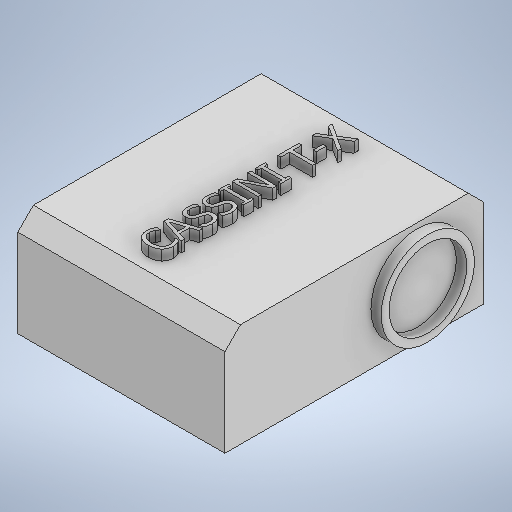
# Autodesk Inventor part: Caméra
Saved by Autodesk Inventor 2026.2 (Build 302298010, 298A)
## iProperties
Created: 2026-04-02
Part Number: Caméra
Material: Générique
Document SubType Name: Modeling
Designer: Genon
Density: 1 g/cm^3
Appearance: Par défaut
Author: Genon
Autodesk Inventor part; units mm, degrees
ref_plane "YZ Plane" through (0, 0, 0) normal (1, 0, 0) x (0, 1, 0)
ref_plane "XZ Plane" through (0, 0, 0) normal (0, 1, 0) x (-1, 0, 0)
ref_plane "XY Plane" through (0, 0, 0) normal (0, 0, 1) x (1, 0, 0)
sketch "Esquisse1" plane through (0, 0, 0) normal (0, 1, 0) x (-1, 0, 0)
  line L0 (0, 0) -> (40, 0)
  line L1 (40, 0) -> (40, -50)
  line L2 (40, -50) -> (0, -50)
  line L3 (0, -50) -> (0, 0)
  dimension "d0" = 40
  dimension "d1" = 50
  constraints: 8 end point, 2 parallel, 1 horizontal, 1 perpendicular
  measures "d0" distance of L1.end L2.end
  measures "d1" distance of L0.end L1.end
extrude "Extrusion1" add sketch "Esquisse1" along normal blind 20
chamfer "Chanfrein1" distance 3 angle 45 2 edges at (-20, 20, 0) (-20, 20, -50)
sketch "Esquisse2" plane through (0, 0, 0) normal (1, 0, 0) x (0, 0, -1)
  circle A0 centre (37.194, 10) radius 7.5
  circle A1 centre (37.194, 10) radius 9
  line L0 (47, 20) -> (3, 20) projected
  line L1 (37.194, 20) -> (37.194, 10)
  line L2 (37.194, 20) -> (47.194, 20) construction
  point P0 (0, 0)
  dimension "d7" = 15
  dimension "d8" = 18
  dimension "d9" = 10
  dimension "d10" = 90
  constraints: 4 end point, 2 centre point, 2 coincident, 2 perpendicular, 1 horizontal, 1 point on line
  measures "d7" diameter of A0
  measures "d8" diameter of A1
  measures "d9" distance of L1.start L1.end
  measures "d10" angle of L1 L2
extrude "Extrusion2" add sketch "Esquisse2" along normal blind 2
sketch "Esquisse6" plane through (0, 20, 0) normal (0, 1, 0) x (1, 0, 0)
  line L0 (-40, 0) -> (0, 0) projected
  line L1 (-40, 50) -> (-40, 0) projected
  line L2 (-22.8083, 5.1679) -> (-22.8083, 50.1014) construction
  line L3 (-22.8083, 50.1014) -> (-1.7313, 50.1014) construction
  line L4 (-1.7313, 50.1014) -> (-1.7313, 5.1679) construction
  line L5 (-1.7313, 5.1679) -> (-22.8083, 5.1679) construction
  spline S0 degree 2 poles (-17.6301, 7.6274) (-17.6301, 7.1411) (-17.9583, 6.3186) (-18.2865, 6.0188) knots 0 0 0 1 2 2 2
  spline S1 degree 2 poles (-18.2865, 6.0188) (-18.6106, 5.7189) (-19.5831, 5.3907) (-20.2152, 5.3907) knots 0 0 0 1 2 2 2
  spline S2 degree 2 poles (-20.2152, 5.3907) (-20.8432, 5.3907) (-21.7751, 5.7108) (-22.1195, 6.0147) knots 0 0 0 1 2 2 2
  spline S3 degree 2 poles (-22.1195, 6.0147) (-22.4558, 6.3146) (-22.8083, 7.133) (-22.8083, 7.6395) knots 0 0 0 1 2 2 2
  spline S4 degree 2 poles (-22.8083, 7.6395) (-22.8083, 7.8907) (-22.7354, 8.3324) (-22.6787, 8.5188) knots 0 0 0 1 2 2 2
  spline S5 degree 2 poles (-22.6787, 8.5188) (-22.626, 8.6808) (-22.4761, 9.0171) (-22.387, 9.1833) knots 0 0 0 1 2 2 2
  line L6 (-22.387, 9.1833) -> (-21.5847, 9.1833)
  line L7 (-21.5847, 9.1833) -> (-21.5847, 9.1306)
  spline S6 degree 2 poles (-21.5847, 9.1306) (-21.6657, 9.0415) (-21.8926, 8.7659) (-22.002, 8.5674) knots 0 0 0 1 2 2 2
  spline S7 degree 2 poles (-22.002, 8.5674) (-22.1074, 8.3769) (-22.2411, 7.9272) (-22.2411, 7.6355) knots 0 0 0 1 2 2 2
  spline S8 degree 2 poles (-22.2411, 7.6355) (-22.2411, 7.3154) (-21.9777, 6.744) (-21.7265, 6.5293) knots 0 0 0 1 2 2 2
  spline S9 degree 2 poles (-21.7265, 6.5293) (-21.4712, 6.3186) (-20.6973, 6.0836) (-20.2152, 6.0836) knots 0 0 0 1 2 2 2
  spline S10 degree 2 poles (-20.2152, 6.0836) (-19.7006, 6.0836) (-18.9591, 6.3308) (-18.7038, 6.5455) knots 0 0 0 1 2 2 2
  spline S11 degree 2 poles (-18.7038, 6.5455) (-18.4566, 6.7562) (-18.2054, 7.3194) (-18.2054, 7.6355) knots 0 0 0 1 2 2 2
  spline S12 degree 2 poles (-18.2054, 7.6355) (-18.2054, 7.9231) (-18.3472, 8.4134) (-18.4526, 8.6039) knots 0 0 0 1 2 2 2
  spline S13 degree 2 poles (-18.4526, 8.6039) (-18.5579, 8.7862) (-18.7767, 9.0577) (-18.8537, 9.1346) knots 0 0 0 1 2 2 2
  line L8 (-18.8537, 9.1346) -> (-18.8537, 9.1833)
  line L9 (-18.8537, 9.1833) -> (-18.0596, 9.1833)
  spline S14 degree 2 poles (-18.0596, 9.1833) (-17.9826, 9.0171) (-17.8408, 8.7254) (-17.7759, 8.5188) knots 0 0 0 1 2 2 2
  spline S15 degree 2 poles (-17.7759, 8.5188) (-17.703, 8.3) (-17.6301, 7.9272) (-17.6301, 7.6274) knots 0 0 0 1 2 2 2
  line L10 (-17.7192, 9.2643) -> (-22.7192, 10.9499)
  line L11 (-22.7192, 10.9499) -> (-22.7192, 11.7684)
  line L12 (-22.7192, 11.7684) -> (-17.7192, 13.4539)
  line L13 (-17.7192, 13.4539) -> (-17.7192, 12.753)
  line L14 (-17.7192, 12.753) -> (-19.1171, 12.2992)
  line L15 (-19.1171, 12.2992) -> (-19.1171, 10.3907)
  line L16 (-19.1171, 10.3907) -> (-17.7192, 9.9369)
  line L17 (-17.7192, 9.9369) -> (-17.7192, 9.2643)
  line L18 (-19.6844, 12.1168) -> (-22.0385, 11.3429)
  line L19 (-22.0385, 11.3429) -> (-19.6844, 10.5731)
  line L20 (-19.6844, 10.5731) -> (-19.6844, 12.1168)
  spline S16 degree 2 poles (-17.6301, 15.3218) (-17.6301, 14.7789) (-17.857, 14.0171) (-18.019, 13.6808) knots 0 0 0 1 2 2 2
  line L21 (-18.019, 13.6808) -> (-18.8537, 13.6808)
  line L22 (-18.8537, 13.6808) -> (-18.8537, 13.7295)
  spline S17 degree 2 poles (-18.8537, 13.7295) (-18.5458, 14.0577) (-18.2054, 14.8883) (-18.2054, 15.2732) knots 0 0 0 1 2 2 2
  spline S18 degree 2 poles (-18.2054, 15.2732) (-18.2054, 15.8243) (-18.6633, 16.3875) (-19.0401, 16.3875) knots 0 0 0 1 2 2 2
  spline S19 degree 2 poles (-19.0401, 16.3875) (-19.3399, 16.3875) (-19.7127, 16.0917) (-19.8059, 15.7716) knots 0 0 0 1 2 2 2
  spline S20 degree 2 poles (-19.8059, 15.7716) (-19.8707, 15.5406) (-19.9599, 15.1557) (-20.0328, 14.868) knots 0 0 0 1 2 2 2
  spline S21 degree 2 poles (-20.0328, 14.868) (-20.1017, 14.6087) (-20.3083, 14.1995) (-20.4745, 14.0415) knots 0 0 0 1 2 2 2
  spline S22 degree 2 poles (-20.4745, 14.0415) (-20.6406, 13.8875) (-21.0863, 13.7173) (-21.378, 13.7173) knots 0 0 0 1 2 2 2
  spline S23 degree 2 poles (-21.378, 13.7173) (-21.9858, 13.7173) (-22.8083, 14.6654) (-22.8083, 15.3988) knots 0 0 0 1 2 2 2
  spline S24 degree 2 poles (-22.8083, 15.3988) (-22.8083, 15.8202) (-22.6422, 16.5658) (-22.4842, 16.8859) knots 0 0 0 1 2 2 2
  line L23 (-22.4842, 16.8859) -> (-21.69, 16.8859)
  line L24 (-21.69, 16.8859) -> (-21.69, 16.8372)
  spline S25 degree 2 poles (-21.69, 16.8372) (-21.9088, 16.5982) (-22.233, 15.8526) (-22.233, 15.4434) knots 0 0 0 1 2 2 2
  spline S26 degree 2 poles (-22.233, 15.4434) (-22.233, 14.9815) (-21.7994, 14.4102) (-21.4469, 14.4102) knots 0 0 0 1 2 2 2
  spline S27 degree 2 poles (-21.4469, 14.4102) (-21.1309, 14.4102) (-20.754, 14.7465) (-20.669, 15.0625) knots 0 0 0 1 2 2 2
  spline S28 degree 2 poles (-20.669, 15.0625) (-20.6122, 15.2732) (-20.4664, 15.8851) (-20.4056, 16.0876) knots 0 0 0 1 2 2 2
  spline S29 degree 2 poles (-20.4056, 16.0876) (-20.2476, 16.6022) (-19.6114, 17.0804) (-19.1455, 17.0804) knots 0 0 0 1 2 2 2
  spline S30 degree 2 poles (-19.1455, 17.0804) (-18.8497, 17.0804) (-18.2824, 16.8413) (-18.0839, 16.6265) knots 0 0 0 1 2 2 2
  spline S31 degree 2 poles (-18.0839, 16.6265) (-17.8651, 16.3875) (-17.6301, 15.7797) (-17.6301, 15.3218) knots 0 0 0 1 2 2 2
  spline S32 degree 2 poles (-17.6301, 19.1509) (-17.6301, 18.6079) (-17.857, 17.8462) (-18.019, 17.5099) knots 0 0 0 1 2 2 2
  line L25 (-18.019, 17.5099) -> (-18.8537, 17.5099)
  line L26 (-18.8537, 17.5099) -> (-18.8537, 17.5585)
  spline S33 degree 2 poles (-18.8537, 17.5585) (-18.5458, 17.8867) (-18.2054, 18.7173) (-18.2054, 19.1022) knots 0 0 0 1 2 2 2
  spline S34 degree 2 poles (-18.2054, 19.1022) (-18.2054, 19.6533) (-18.6633, 20.2165) (-19.0401, 20.2165) knots 0 0 0 1 2 2 2
  spline S35 degree 2 poles (-19.0401, 20.2165) (-19.3399, 20.2165) (-19.7127, 19.9207) (-19.8059, 19.6006) knots 0 0 0 1 2 2 2
  spline S36 degree 2 poles (-19.8059, 19.6006) (-19.8707, 19.3697) (-19.9599, 18.9847) (-20.0328, 18.697) knots 0 0 0 1 2 2 2
  spline S37 degree 2 poles (-20.0328, 18.697) (-20.1017, 18.4377) (-20.3083, 18.0285) (-20.4745, 17.8705) knots 0 0 0 1 2 2 2
  spline S38 degree 2 poles (-20.4745, 17.8705) (-20.6406, 17.7165) (-21.0863, 17.5463) (-21.378, 17.5463) knots 0 0 0 1 2 2 2
  spline S39 degree 2 poles (-21.378, 17.5463) (-21.9858, 17.5463) (-22.8083, 18.4945) (-22.8083, 19.2278) knots 0 0 0 1 2 2 2
  spline S40 degree 2 poles (-22.8083, 19.2278) (-22.8083, 19.6492) (-22.6422, 20.3948) (-22.4842, 20.7149) knots 0 0 0 1 2 2 2
  line L27 (-22.4842, 20.7149) -> (-21.69, 20.7149)
  line L28 (-21.69, 20.7149) -> (-21.69, 20.6663)
  spline S41 degree 2 poles (-21.69, 20.6663) (-21.9088, 20.4272) (-22.233, 19.6817) (-22.233, 19.2724) knots 0 0 0 1 2 2 2
  spline S42 degree 2 poles (-22.233, 19.2724) (-22.233, 18.8105) (-21.7994, 18.2392) (-21.4469, 18.2392) knots 0 0 0 1 2 2 2
  spline S43 degree 2 poles (-21.4469, 18.2392) (-21.1309, 18.2392) (-20.754, 18.5755) (-20.669, 18.8915) knots 0 0 0 1 2 2 2
  spline S44 degree 2 poles (-20.669, 18.8915) (-20.6122, 19.1022) (-20.4664, 19.7141) (-20.4056, 19.9167) knots 0 0 0 1 2 2 2
  spline S45 degree 2 poles (-20.4056, 19.9167) (-20.2476, 20.4312) (-19.6114, 20.9094) (-19.1455, 20.9094) knots 0 0 0 1 2 2 2
  spline S46 degree 2 poles (-19.1455, 20.9094) (-18.8497, 20.9094) (-18.2824, 20.6703) (-18.0839, 20.4556) knots 0 0 0 1 2 2 2
  spline S47 degree 2 poles (-18.0839, 20.4556) (-17.8651, 20.2165) (-17.6301, 19.6087) (-17.6301, 19.1509) knots 0 0 0 1 2 2 2
  line L29 (-17.7192, 23.3283) -> (-17.7192, 21.3915)
  line L30 (-17.7192, 21.3915) -> (-18.2297, 21.3915)
  line L31 (-18.2297, 21.3915) -> (-18.2297, 22.0277)
  line L32 (-18.2297, 22.0277) -> (-22.2087, 22.0277)
  line L33 (-22.2087, 22.0277) -> (-22.2087, 21.3915)
  line L34 (-22.2087, 21.3915) -> (-22.7192, 21.3915)
  line L35 (-22.7192, 21.3915) -> (-22.7192, 23.3283)
  line L36 (-22.7192, 23.3283) -> (-22.2087, 23.3283)
  line L37 (-22.2087, 23.3283) -> (-22.2087, 22.6922)
  line L38 (-22.2087, 22.6922) -> (-18.2297, 22.6922)
  line L39 (-18.2297, 22.6922) -> (-18.2297, 23.3283)
  line L40 (-18.2297, 23.3283) -> (-17.7192, 23.3283)
  line L41 (-17.7192, 27.7287) -> (-17.7192, 26.9831)
  line L42 (-17.7192, 26.9831) -> (-22.0304, 24.7708)
  line L43 (-22.0304, 24.7708) -> (-17.7192, 24.7708)
  line L44 (-17.7192, 24.7708) -> (-17.7192, 24.1509)
  line L45 (-17.7192, 24.1509) -> (-22.7192, 24.1509)
  line L46 (-22.7192, 24.1509) -> (-22.7192, 25.0949)
  line L47 (-22.7192, 25.0949) -> (-18.7605, 27.1087)
  line L48 (-18.7605, 27.1087) -> (-22.7192, 27.1087)
  line L49 (-22.7192, 27.1087) -> (-22.7192, 27.7287)
  line L50 (-22.7192, 27.7287) -> (-17.7192, 27.7287)
  line L51 (-17.7192, 30.4839) -> (-17.7192, 28.5471)
  line L52 (-17.7192, 28.5471) -> (-18.2297, 28.5471)
  line L53 (-18.2297, 28.5471) -> (-18.2297, 29.1833)
  line L54 (-18.2297, 29.1833) -> (-22.2087, 29.1833)
  line L55 (-22.2087, 29.1833) -> (-22.2087, 28.5471)
  line L56 (-22.2087, 28.5471) -> (-22.7192, 28.5471)
  line L57 (-22.7192, 28.5471) -> (-22.7192, 30.4839)
  line L58 (-22.7192, 30.4839) -> (-22.2087, 30.4839)
  line L59 (-22.2087, 30.4839) -> (-22.2087, 29.8478)
  line L60 (-22.2087, 29.8478) -> (-18.2297, 29.8478)
  line L61 (-18.2297, 29.8478) -> (-18.2297, 30.4839)
  line L62 (-18.2297, 30.4839) -> (-17.7192, 30.4839)
  line L63 (-17.7192, 34.6209) -> (-22.1276, 34.6209)
  line L64 (-22.1276, 34.6209) -> (-22.1276, 32.9434)
  line L65 (-22.1276, 32.9434) -> (-22.7192, 32.9434)
  line L66 (-22.7192, 32.9434) -> (-22.7192, 36.9628)
  line L67 (-22.7192, 36.9628) -> (-22.1276, 36.9628)
  line L68 (-22.1276, 36.9628) -> (-22.1276, 35.2854)
  line L69 (-22.1276, 35.2854) -> (-17.7192, 35.2854)
  line L70 (-17.7192, 35.2854) -> (-17.7192, 34.6209)
  line L71 (-19.6033, 39.159) -> (-19.6033, 37.2667)
  line L72 (-19.6033, 37.2667) -> (-20.2111, 37.2667)
  line L73 (-20.2111, 37.2667) -> (-20.2111, 39.159)
  line L74 (-20.2111, 39.159) -> (-19.6033, 39.159)
  line L75 (-17.7192, 43.4215) -> (-17.7192, 42.6598)
  line L76 (-17.7192, 42.6598) -> (-19.7127, 41.4442)
  line L77 (-19.7127, 41.4442) -> (-17.7192, 40.2043)
  line L78 (-17.7192, 40.2043) -> (-17.7192, 39.4872)
  line L79 (-17.7192, 39.4872) -> (-20.2233, 41.0795)
  line L80 (-20.2233, 41.0795) -> (-22.7192, 39.5358)
  line L81 (-22.7192, 39.5358) -> (-22.7192, 40.2975)
  line L82 (-22.7192, 40.2975) -> (-20.7622, 41.4888)
  line L83 (-20.7622, 41.4888) -> (-22.7192, 42.7043)
  line L84 (-22.7192, 42.7043) -> (-22.7192, 43.4215)
  line L85 (-22.7192, 43.4215) -> (-20.2557, 41.8575)
  line L86 (-20.2557, 41.8575) -> (-17.7192, 43.4215)
  constraints: 2 other
extrude "Extrusion5" add sketch "Esquisse6" along normal blind 2
sketch "Esquisse7" plane through (0, 0, 0) normal (0, -1, 0) x (1, 0, 0)
  line L0 (0, 0) -> (0, -25)
  line L1 (0, -25) -> (-20, -25)
  line L2 (-35, -10) -> (-5, -10)
  line L3 (-5, -10) -> (-5, -40)
  line L4 (-5, -40) -> (-35, -40)
  line L5 (-35, -40) -> (-35, -10)
  line L6 (-35, -10) -> (-5, -40) construction
  line L7 (-5, -10) -> (-35, -40) construction
  dimension "d39" = 25
  dimension "d40" = 20
  dimension "d41" = 30
  dimension "d42" = 30
  constraints: 16 end point, 2 midpoint, 2 parallel, 2 perpendicular, 1 horizontal, 1 vertical
  measures "d39" distance of L0.start L0.end
  measures "d40" distance of L0.end L1.end
  measures "d41" distance of L3.end L4.end
  measures "d42" distance of L2.end L3.end
extrude "Extrusion6" cut sketch "Esquisse7" against normal blind 3
sketch "Esquisse8" plane through (0, 3, 0) normal (0, -1, 0) x (1, 0, 0)
  line L0 (0, 0) -> (0, -3) projected
  line L1 (0, 0) -> (0, -25)
  line L2 (0, -25) -> (-20, -25)
  line L3 (-30, -15) -> (-10, -15)
  line L4 (-10, -15) -> (-10, -35)
  line L5 (-10, -35) -> (-30, -35)
  line L6 (-30, -35) -> (-30, -15)
  line L7 (-30, -15) -> (-10, -35) construction
  line L8 (-10, -15) -> (-30, -35) construction
  dimension "d45" = 25
  dimension "d46" = 20
  dimension "d47" = 20
  dimension "d48" = 20
  constraints: 16 end point, 2 midpoint, 2 parallel, 2 perpendicular, 1 collinear, 1 horizontal
  measures "d45" distance of L0.start L1.end
  measures "d46" distance of L1.end L2.end
  measures "d47" distance of L4.end L5.end
  measures "d48" distance of L3.end L4.end
extrude "Extrusion7" cut sketch "Esquisse8" against normal blind 12
sketch "Esquisse9" plane through (-10, 3, -15) normal (0, 0, -1) x (-1, 0, 0)
  line L0 (0, 0) -> (0, 12) projected
  line L1 (0, 0) -> (0, 2)
  line L2 (0, 2) -> (20, 2)
  line L3 (20, 2) -> (20, 12)
  line L4 (20, 12) -> (0, 12)
  line L5 (0, 12) -> (0, 2)
  point P0 (-10, -3)
  dimension "d51" = 2
  dimension "d52" = 20
  constraints: 10 end point, 2 parallel, 1 horizontal, 1 perpendicular, 1 point on line
  measures "d51" distance of L0.start L1.end
  measures "d52" distance of L4.end L3.end
extrude "Extrusion8" cut sketch "Esquisse9" against normal blind 10
sketch "Esquisse10" plane through (-30, 3, -35) normal (0, 0, 1) x (1, 0, 0)
  line L0 (25, 0) -> (-5, 0) projected
  line L1 (25, 0) -> (20, 0)
  line L2 (20, 0) -> (20, 2)
  line L3 (20, 2) -> (0, 2)
  line L4 (0, 2) -> (0, 12)
  line L5 (0, 12) -> (20, 12)
  line L6 (20, 12) -> (20, 2)
  point P0 (30, -3)
  dimension "d55" = 5
  dimension "d56" = 2
  dimension "d57" = 20
  dimension "d58" = 10
  constraints: 12 end point, 2 parallel, 1 horizontal, 1 perpendicular, 1 point on line, 1 vertical
  measures "d55" distance of L0.start L1.end
  measures "d56" distance of L1.end L2.end
  measures "d57" distance of L4.end L5.end
  measures "d58" distance of L3.end L4.end
extrude "Extrusion9" cut sketch "Esquisse10" against normal blind 10
